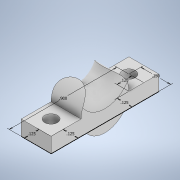
# Autodesk Inventor part: DualSensorReadout - CableClamp
Saved by Autodesk Inventor 2020 (Build 240168000, 168)
## iProperties
Created: 2024-01-28
Part Number: DualSensorReadout - CableClamp
Material: Generic
Document SubType Name: Modeling
Designer: Beaucage
Density: 1 g/cm^3
Appearance: Default
Author: Beaucage
Autodesk Inventor part; units mm, degrees
ref_plane "YZ Plane" through (0, 0, 0) normal (1, 0, 0) x (0, 1, 0)
ref_plane "XZ Plane" through (0, 0, 0) normal (0, 1, 0) x (-1, 0, 0)
ref_plane "XY Plane" through (0, 0, 0) normal (0, 0, 1) x (1, 0, 0)
sketch "Sketch1" plane through (0, 0, 0) normal (0, 1, 0) x (-1, 0, 0)
  line L0 (0, 0) -> (6.35, 0)
  line L1 (6.35, 0) -> (6.35, -22.86)
  line L2 (6.35, -22.86) -> (0, -22.86)
  line L3 (0, -22.86) -> (0, 0)
  line L4 (0, 0) -> (3.175, 0)
  line L5 (3.175, 0) -> (3.175, -3.175)
  line L6 (3.175, -3.175) -> (0, -3.175)
  line L7 (0, -3.175) -> (0, 0)
  line L8 (0, -22.86) -> (3.175, -22.86)
  line L9 (3.175, -22.86) -> (3.175, -19.685)
  line L10 (3.175, -19.685) -> (0, -19.685)
  line L11 (0, -19.685) -> (0, -22.86)
  dimension "d0" = 6.35
  dimension "d1" = 22.86
  dimension "d2" = 3.175
  dimension "d3" = 3.175
  dimension "d4" = 3.175
  dimension "d5" = 3.175
  constraints: 24 end point, 6 parallel, 3 horizontal, 3 perpendicular
  measures "d0" distance of L1.end L2.end
  measures "d1" distance of L0.end L1.end
  measures "d2" distance of L5.end L6.end
  measures "d3" distance of L4.end L5.end
  measures "d4" distance of L10.end L9.end
  measures "d5" distance of L9.end L8.end
extrude "Extrusion1" add sketch "Sketch1" along normal blind 3.175
hole "Hole1" at (-3.175, 0, -3.175) at (-3.175, 0, -19.685) direction (0, 1, 0) diameter 2.7051 depth 6.35
sketch "Sketch2" plane through (0, 0, 0) normal (1, 0, 0) x (0, 0, -1)
  line L0 (0, 3.175) -> (22.86, 3.175) projected
  circle A0 centre (11.43, 3.175) radius 5.08
  circle A1 centre (11.43, 8.255) radius 2.54
  point P0 (0, 0)
  point P1 (13.8893, 7.62)
  point P2 (8.9707, 7.62)
  point P3 (6.35, 3.175)
  point P4 (16.51, 3.175)
  dimension "d15" = 10.16
  dimension "d16" = 5.08
  constraints: 1 centre point, 1 midpoint, 3 other
  measures "d16" diameter of A1
extrude "Extrusion2" add sketch "Sketch2" against normal blind 6.35 contours A0 A1 L0 | L0 A0
fillet "Fillet1" radius 3.175 2 edges at (0, 5.715, -11.43) (-6.35, 5.715, -11.43)
body "Solid1"
